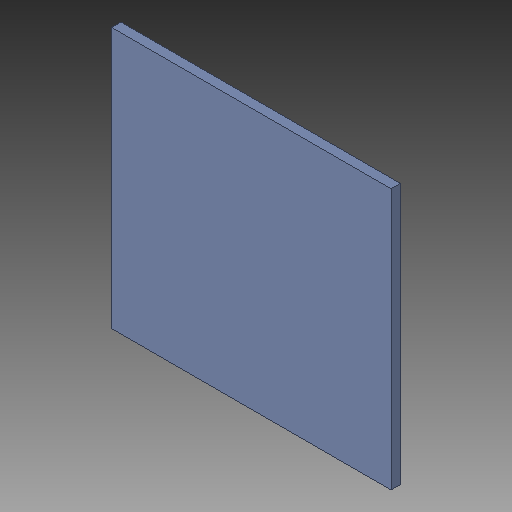
# Autodesk Inventor part: GBX_005.1-fence-plate
Saved by Autodesk Inventor 2019 (Build 230136000, 136)
## iProperties
Created: 2019-08-15
Part Number: GBX_005.1-fence-plate
Material: Generic
Document SubType Name: Modeling
Designer: Rene
Density: 1 g/cm^3
Appearance: Rubber - Blue
Author: Rene
Autodesk Inventor part; units mm, degrees
ref_plane "YZ Plane" through (0, 0, 0) normal (1, 0, 0) x (0, 1, 0)
ref_plane "XZ Plane" through (0, 0, 0) normal (0, 1, 0) x (-1, 0, 0)
ref_plane "XY Plane" through (0, 0, 0) normal (0, 0, 1) x (1, 0, 0)
sketch "Sketch1" plane through (0, 0, 0) normal (0, 0, 1) x (1, 0, 0)
  line L0 (150, -140) -> (-150, -140)
  line L1 (-150, -140) -> (-150, 140)
  line L2 (-150, 140) -> (150, 140)
  line L3 (150, 140) -> (150, -140)
  line L4 (150, -140) -> (-150, 140) construction
  line L5 (-150, -140) -> (150, 140) construction
  point P0 (0, 0)
  dimension "d0" = 280
  dimension "d1" = 300
  constraints: 12 end point, 2 midpoint, 2 parallel, 1 horizontal, 1 perpendicular
  measures "d0" distance of L0.end L1.end
  measures "d1" distance of L1.end L2.end
extrude "Extrusion1" add sketch "Sketch1" along normal blind 10
body "Solid1"
